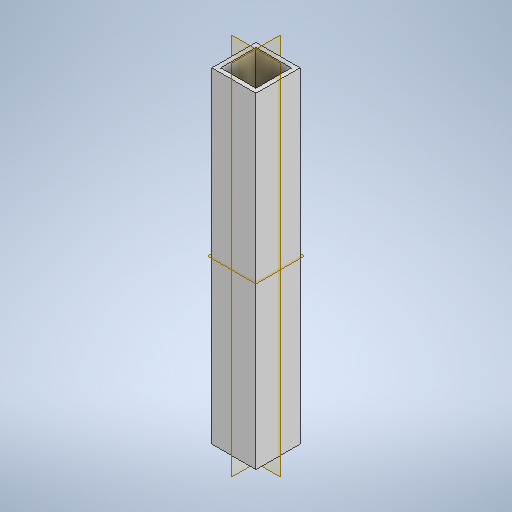
# Autodesk Inventor part: Perna para Exercício
Saved by Autodesk Inventor 2025.2 (Build 292293000, 293)
## iProperties
Created: 2025-04-07
Part Number: Perna para Exercício
Material: Genérico
Document SubType Name: Sheet Metal
Designer: kenay
Density: 1 g/cm^3
Sheet Metal Rule: Padrão_mm
Appearance: Padrão
Author: kenay
Autodesk Inventor part; units mm, degrees
sketch "Esboço1" plane through (0, 0, 0) normal (0, 1, 0) x (-1, 0, 0)
  line L0 (-50, 50) -> (50, 50)
  line L1 (50, 50) -> (50, -50)
  line L2 (50, -50) -> (-50, -50)
  line L3 (-50, -50) -> (-50, 50)
  line L4 (-50, 50) -> (50, -50) construction
  line L5 (50, 50) -> (-50, -50) construction
  line L6 (-40, 40) -> (40, 40)
  line L7 (40, 40) -> (40, -40)
  line L8 (40, -40) -> (-40, -40)
  line L9 (-40, -40) -> (-40, 40)
  line L10 (-40, 40) -> (40, -40) construction
  line L11 (40, 40) -> (-40, -40) construction
  point P0 (0, 0)
  dimension "d0" = 100
  dimension "d1" = 10
  constraints: 24 end point, 4 midpoint, 4 parallel, 4 perpendicular, 2 horizontal
  measures "d0" distance of L1.end L2.end
  measures "d1" distance between parallel lines of L2 L8
extrude "Extrusão1" add sketch "Esboço1" along normal mid plane 740
equation "\"Raio_vergadura\" = Espessura"
equation "\"Largura_alívio_de_vergadura\" = Espessura"
equation "\"Profundidade_alívio_de_vergadura\" = 0.5 * Espessura"
equation "\"Tamanho_alívio_de_dobra\" = 4 * Espessura"
equation "\"Remanescente_mínimo\" = 2 * Espessura"
equation "\"Raiodetransição\" = Raio_vergadura"
equation "\"Tamanho_de_raio_de_Jacobi\" = Raio_vergadura"
equation "\"TamanhoFolga\" = Espessura"
equation "\"Espessura\" = 0.5"
